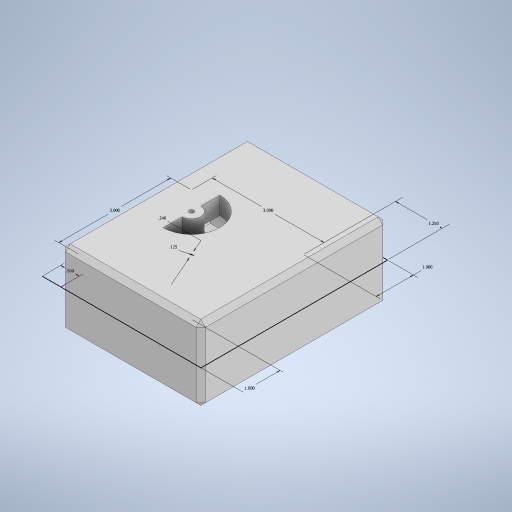
# Autodesk Inventor part: Flywheel Cutting Jig
Saved by Autodesk Inventor 2023 (Build 270158000, 158)
## iProperties
Created: 2022-12-31
Part Number: Flywheel Cutting Jig
Material: Generic
Document SubType Name: Modeling
Designer: tgr41
Density: 1 g/cm^3
Appearance: Default
Author: tgr41
Autodesk Inventor part; units mm, degrees
ref_plane "YZ Plane" through (0, 0, 0) normal (1, 0, 0) x (0, 1, 0)
ref_plane "XZ Plane" through (0, 0, 0) normal (0, 1, 0) x (-1, 0, 0)
ref_plane "XY Plane" through (0, 0, 0) normal (0, 0, 1) x (1, 0, 0)
sketch "Sketch1" plane through (0, 0, 0) normal (0, 1, 0) x (-1, 0, 0)
  line L0 (0, 0) -> (76.2, 0)
  line L1 (76.2, 0) -> (76.2, -76.2)
  line L2 (76.2, -76.2) -> (0, -76.2)
  line L3 (0, -76.2) -> (0, 0)
  line L4 (-31.7621, 25.4) -> (76.2, 25.4)
  line L5 (76.2, -101.6) -> (-31.7621, -101.6)
  line L6 (-31.7621, -101.6) -> (-31.7621, 25.4)
  line L7 (76.2, 25.4) -> (63.5, 25.4)
  line L8 (63.5, 25.4) -> (63.5, -101.6)
  line L9 (76.2, -38.1) -> (0, -38.1)
  line L10 (38.1, 0) -> (38.1, -76.2)
  circle A0 centre (38.1, -38.1) radius 3.048
  circle A1 centre (38.1, -38.1) radius 1.5875
  circle A2 centre (38.1, -38.1) radius 6.3171
  circle A3 centre (38.1, -38.1) radius 19.2182
  point P0 (63.5, 0)
  point P1 (63.5, -76.2)
  point P2 (38.1, -57.3182)
  point P3 (38.1, -44.4171)
  point P4 (38.1, -31.7829)
  point P5 (38.1, -18.8818)
  dimension "d0" = 76.2
  dimension "d1" = 76.2
  dimension "d2" = 25.4
  dimension "d3" = 25.4
  dimension "d4" = 31.7621
  dimension "d6" = 12.7
  dimension "d7" = 6.096
  dimension "d12" = 3.175
  constraints: 22 end point, 5 midpoint, 4 centre point, 3 coincident, 3 parallel, 2 horizontal, 2 perpendicular, 2 point on line
  measures "d0" distance of L1.end L2.end
  measures "d1" distance of L0.end L1.end
  measures "d2" distance between parallel lines of L5 L2
  measures "d3" distance between parallel lines of L4 L0
  measures "d4" distance between parallel lines of L6 L3
  measures "d6" distance of L4.end L7.end
  measures "d7" diameter of A0
  measures "d12" diameter of A1
extrude "Extrusion1" add sketch "Sketch1" along normal mid plane 50.8 contours L3 L2 L8 L5 L6 L4 L0 | L0 L10 A3 L9 L3 | L0 L8 L9 A3 L10 | L9 A3 L10 L2 L3 | A3 L9 A2 L10 | L10 A2 L9 A3 | L9 A2 L10 A3 | L8 L2 L10 A3 L9 | A2 L9 A0 L10 | L10 A0 L9 A2 | A3 L10 A2 L9 | L9 A0 L10 A2 | A0 L9 A1 L10 | L10 A1 L9 A0 | A2 L10 A0 L9 | L9 A1 L10 A0 | A1 L9 L10 | L10 L9 A1 | A0 L10 A1 L9 | L9 L10 A1 | L9 A1 L10
extrude "Extrusion2" cut sketch "Sketch1" along normal mid plane 26.67 contours L0 L10 A3 L9 L3 | L0 L8 L9 A3 L10 | L9 A3 L10 L2 L3 | A3 L9 A2 L10 | L10 A2 L9 A3 | L9 A2 L10 A3 | L8 L2 L10 A3 L9 | A2 L9 A0 L10 | L10 A0 L9 A2 | A3 L10 A2 L9 | L9 A0 L10 A2 | A0 L9 A1 L10 | L10 A1 L9 A0 | A2 L10 A0 L9 | L9 A1 L10 A0 | A1 L9 L10 | L10 L9 A1 | A0 L10 A1 L9 | L9 L10 A1 | L9 A1 L10
extrude "Extrusion3" cut sketch "Sketch1" along normal blind 26.67 contours A1 L9 L10 | L10 L9 A1 | L9 L10 A1 | L9 A1 L10
extrude "Extrusion4" cut sketch "Sketch1" against normal blind 26.67 contours A0 L9 A1 L10 | L10 A1 L9 A0 | L9 A1 L10 A0 | A1 L9 L10 | L10 L9 A1 | A0 L10 A1 L9 | L9 L10 A1 | L9 A1 L10
extrude "Extrusion5" cut sketch "Sketch1" along normal mid plane 76.2 contours L10 A2 L9 A3 | L9 A2 L10 A3 picked at (24.03, -33.4265) picked at (23.3428, -39.5255)
chamfer "Chamfer1" distance 3.175 angle 45 12 edges at (31.7621, -25.4, -38.1) (31.7621, 0, -101.6) (31.7621, 25.4, -38.1) (31.7621, 0, 25.4) (-15.8689, -25.4, 25.4) (-15.8689, -25.4, -101.6) (-15.8689, 25.4, 25.4) (-15.8689, 25.4, -101.6) (-63.5, 0, -101.6) (-63.5, 25.4, -38.1) (-63.5, 0, 25.4) (-63.5, -25.4, -38.1)
body "Solid1"
